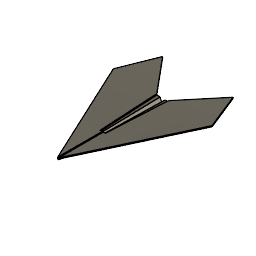
Paper Rocket-2 (Autodesk Fusion 360 design; units mm, degrees)
part number: 2026-08-13-23-00-56-069
Autodesk Fusion 360 part; units mm, degrees
sketch "Sketch1" plane through (0, 0, 0) normal (0, 0, 1) x (1, 0, 0)
  line L0 (0.7014, -148.4969) -> (70, 0)
  line L1 (70, 0) -> (50, 50)
  line L2 (50, 50) -> (8.3707, 0)
  line L3 (-50, 50) -> (-8.3707, 0)
  line L4 (-70, 0) -> (-50, 50)
  line L5 (-0.7014, -148.4969) -> (-70, 0)
  line L6 (-3.6273, -85) -> (3.6273, -85)
  line L7 (-8.3707, 0) -> (-3.6273, -85)
  line L8 (0, 225) -> (0, -85)
  line L9 (8.3707, 0) -> (3.6273, -85)
  line L10 (-0.7014, -148.4969) -> (0.7014, -148.4969)
  constraint vertical L8
  constraint symmetric L0.end L4.start L8
  constraint symmetric L1.end L3.start L8
  constraint symmetric L2.end L3.end L8
  constraint perpendicular L6 L8
  constraint coincident L6 L8.end
  constraint horizontal L10
extrude "Extrude1" add sketch "Sketch1" along normal blind 1.5 makes body 1
sketch "Sketch2" plane through (0, 0, 0) normal (0, 1, 0) x (1, 0, 0)
  line L0 (0, 10) -> (-3.6, 0)
  line L1 (-3.6, 0) -> (-12, 0)
  line L2 (-12, 0) -> (0, 25)
  line L3 (0, -6) -> (0, 31)
  line L4 (0, 10) -> (3.6, 0)
  line L5 (3.6, 0) -> (12, 0)
  line L6 (12, 0) -> (0, 25)
  constraint horizontal L1
  constraint vertical L3
  constraint symmetric L0.start L3 L4.start
  constraint symmetric L0.end L3 L4.end
  constraint symmetric L1.end L3 L5.end
  constraint symmetric L2.end L3 L6.end
sketch "Sketch3" plane through (0, -148.4969, 0) normal (0, -1, 0) x (1, 0, 0)
  line L0 (-0.7014, 0) -> (0.7014, 0)
  line L1 (0.7014, 0) -> (0.7014, 1.5)
  line L2 (0.7014, 1.5) -> (-0.7014, 1.5)
  line L3 (-0.7014, 1.5) -> (-0.7014, 0)
  line L4 (-0.7014, 0) -> (0, -1.5)
  line L5 (0, 6) -> (0, -31)
  line L6 (0.7014, 0) -> (0, -1.5)
  line L7 (-0.7014, 0) -> (0.7014, 0)
  constraint coincident L0.start L3.end
  constraint symmetric L0.start L5 L0.end
loft "Loft1" add profiles "Sketch3", "Sketch2" section 1 contours L0 L4 L5 L7 | L0 L5 L6 L7 section 2 separate body makes body 2
extrude "Extrude2" cut 1 faces at (-0.2338, -148.4969, 0.5) along direction (0, 1, 0) blind 170 on bodies 1 bodies 1 makes body 3 at (27.3327, -28.3333, 0)
